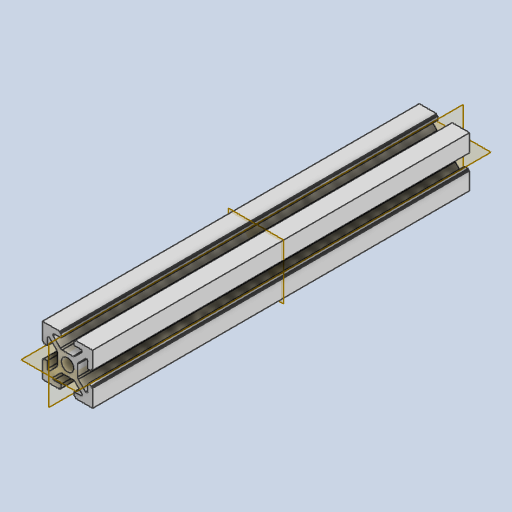
# Autodesk Inventor part: Perfil 20_500
Saved by Autodesk Inventor 2025.2 (Build 292293000, 293)
## iProperties
Created: 2025-03-25
Part Number: Perfil 20_500
Material: Generic
Document SubType Name: Modeling
Designer: ishad
Density: 1 g/cm^3
Appearance: Default
Author: ishad
Autodesk Inventor part; units mm, degrees
sketch "Sketch1" plane through (0, 0, 0) normal (0, 0, 1) x (1, 0, 0)
  line L0 (-10, 10) -> (10, 10) construction
  circle A0 centre (0, 0) radius 2.5 construction
  line L1 (4, 4) -> (-4, 4) construction
  line L2 (0, 0) -> (-10, 10) construction
  line L3 (-2.5858, 4) -> (-6.5858, 8) construction
  line L4 (-10, 10) -> (-4, 4)
  line L5 (-6.5858, 8) -> (-2.5858, 8) construction
  line L6 (-2.5858, 8) -> (-2.5858, 10) construction
  line L7 (-2.5858, 10) -> (-3.0858, 10) construction
  line L8 (-3.0858, 10) -> (-3.0858, 9.5)
  line L9 (-3.0858, 9.5) -> (-2.5858, 9.5)
  line L10 (-2.5858, 9.5) -> (-2.5858, 10) construction
  line L11 (-2.5858, 9.5) -> (-2.5858, 8)
  line L12 (-10, 10) -> (-3.0858, 10)
  line L13 (-4, 4) -> (-4, 0) construction
  line L14 (-10, 10) -> (-16.9142, 10)
  line L15 (0, 4) -> (-2.5858, 4)
  arc A1 (0, 2.5) -> (-1.7678, 1.7678) centre (0, 0) ccw
  line L16 (-4, 4) -> (-1.7678, 1.7678)
  line L17 (0, 4) -> (0, 2.5)
  circle A2 centre (0, 0) radius 2.5 construction
  line L18 (-4, -4) -> (-4, 4) construction
  line L19 (-4, 2.5858) -> (-8, 6.5858) construction
  line L20 (-8, 6.5858) -> (-8, 2.5858) construction
  line L21 (-8, 2.5858) -> (-10, 2.5858) construction
  line L22 (-10, 2.5858) -> (-10, 3.0858) construction
  line L23 (-10, 3.0858) -> (-9.5, 3.0858)
  line L24 (-9.5, 3.0858) -> (-9.5, 2.5858)
  line L25 (-9.5, 2.5858) -> (-10, 2.5858) construction
  line L26 (-9.5, 2.5858) -> (-8, 2.5858)
  line L27 (-10, 10) -> (-10, 3.0858)
  line L28 (-4, 4) -> (0, 4) construction
  line L29 (-10, 10) -> (-10, 16.9142)
  line L30 (-4, 0) -> (-4, 2.5858)
  arc A3 (-1.7678, 1.7678) -> (-2.5, 0) centre (0, 0) ccw
  line L31 (-4, 0) -> (-2.5, 0)
  arc A4 (-5.3787, 8) -> (-5.7322, 7.1464) centre (-5.3787, 7.5) ccw
  arc A5 (-7.1464, 5.7322) -> (-8, 5.3787) centre (-7.5, 5.3787) ccw
  arc A6 (-2.8787, 4.2929) -> (-2.1716, 4) centre (-2.1716, 5) ccw
  arc A7 (-4, 2.1716) -> (-4.2929, 2.8787) centre (-5, 2.1716) ccw
  line L32 (-8, 5.3787) -> (-8, 2.5858)
  line L33 (-7.1464, 5.7322) -> (-4.2929, 2.8787)
  line L34 (-5.7322, 7.1464) -> (-2.8787, 4.2929)
  line L35 (-5.3787, 8) -> (-2.5858, 8)
  point P0 (0, 10)
  point P1 (-10, 0)
  point P2 (-2.1716, 4)
  dimension "d0" = 20
  dimension "d1" = 10
  dimension "d2" = 5
  dimension "d3" = 6
  dimension "d20" = 1
  dimension "d21" = 2
  dimension "d25" = 0.5
  dimension "d38" = 0.5
  dimension "d39" = 1
  constraints: 74 end point, 16 point on circle, 13 point on line, 13 symmetric about line, 8 centre point, 8 tangent, 6 horizontal, 5 collinear, 5 vertical alignment, 3 equal radius, 3 parallel, 3 vertical, 2 equal length, 2 midpoint, 2 perpendicular, 1 coincident, 1 horizontal alignment, 2 other
  measures "d0" distance of L0.start L0.end
  measures "d1" distance from line of point (0, 0) L0
  measures "d2" diameter of A0
  measures "d3" distance between parallel lines of L0 L1
  measures "d20" distance between parallel lines of L2 L3
  measures "d21" distance from line of L0 L3.end
  measures "d25" distance of L8.end L9.end
  measures "d38" radius of A4
  measures "d39" radius of A7
extrude "Extrusion1" add sketch "Sketch1" along normal mid plane 150
mirror "Mirror1" about plane through (0, 0, 0) normal (1, 0, 0) of "Extrusion1"
mirror "Mirror2" about plane through (0, 0, 0) normal (0, 1, 0) of "Extrusion1", "Mirror1"
sketch "Sketch2" plane through (0, 0, 0) normal (0, 0, 1) x (1, 0, 0)
  point P0 (0, 0)
equation "\"d1\" = 0.5 * d0"
body "Solid1"
